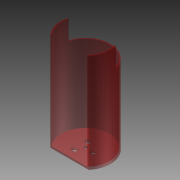
# Autodesk Inventor part: ss_inner_guide_top
Saved by Autodesk Inventor 2011 SP2 (Build 150309200, 309)
## iProperties
Created: 2012-05-22
Part Number: ss_inner_guide_top
Document SubType Name: Modeling
Designer: sungwook
Density: 1 g/cm^3
Author: sungwook
Autodesk Inventor part; units mm, degrees
ref_plane "YZ Plane" through (0, 0, 0) normal (1, 0, 0) x (0, 1, 0)
sketch "Sketch1" plane through (0, 0, 0) normal (0, 0, 1) x (1, 0, 0)
  circle A0 centre (0, 0) radius 12.75
  circle A1 centre (0, 0) radius 12.25
  dimension "d0" = 25.5
  dimension "d1" = 24.5
  constraints: 2 centre point, 2 coincident
  measures "d0" diameter of A0
  measures "d1" diameter of A1
extrude "Extrusion1" add sketch "Sketch1" along normal blind 49.5
sketch "Sketch2" plane through (0, 0, 49.5) normal (0, 0, 1) x (1, 0, 0)
  line L0 (-17.85, 0) -> (17.85, 0) projected
  line L1 (0, -17.85) -> (0, 17.85) projected
  line L2 (0, 0) -> (-12.3156, 3.2999)
  line L3 (0, 0) -> (-9.0156, -9.0156)
  line L4 (0, 0) -> (12.3156, 3.2999)
  line L5 (0, 0) -> (9.0156, -9.0156)
  arc A0 (11.8326, 3.1705) -> (-11.8326, 3.1705) centre (0, 0) ccw
  arc A1 (-8.6621, -8.6621) -> (8.6621, -8.6621) centre (0, 0) ccw
  circle A2 centre (0, 0) radius 12.75 projected
  dimension "d4" = 15
  dimension "d5" = 45
  constraints: 8 end point, 8 point on circle, 4 point on line, 2 centre point, 2 coincident, 2 symmetric about line
  measures "d4" angle of L0 L2
  measures "d5" angle of L3 L0
extrude "Extrusion2" cut sketch "Sketch2" against normal blind 10 contours L5 A1 L1 | L1 A1 L3 | A1 L5 A2 L1 | L1 A2 L3 A1 | A0 L2 A2 L1 | L1 A2 L4 A0
sketch "Sketch3" plane through (0, 0, 0) normal (0, 0, -1) x (-1, 0, 0)
  circle A0 centre (0, 0) radius 12.75 projected
extrude "Extrusion3" add sketch "Sketch3" along normal blind 1
ref_plane "Work Plane1" through (0, -12.75, 0) normal (0, 1, 0) x (-1, 0, 0)
ref_plane "Work Plane2" through (0, -12.75, 0) normal (0, 1, 0) x (-1, 0, 0)
sketch "Sketch7" plane through (0, 0, 49.5) normal (0, 0, 1) x (1, 0, 0)
  arc A0 (9.0156, -9.0156) -> (12.3156, 3.2999) centre (0, 0) ccw projected
  arc A1 (8.6621, -8.6621) -> (11.8326, 3.1705) centre (0, 0) ccw projected
  line L0 (8.6621, -8.6621) -> (9.0156, -9.0156) projected
  line L1 (-10.4211, -8.1317) -> (11.1081, -8.1317)
  line L2 (11.1081, -8.1317) -> (11.1081, -13.0652)
  line L3 (11.1081, -13.0652) -> (-10.4211, -13.0652)
  line L4 (-10.4211, -13.0652) -> (-10.4211, -8.1317)
  constraints: 8 end point, 2 parallel, 1 horizontal, 1 perpendicular
extrude "Extrusion6" cut sketch "Sketch7" against normal through all
sketch "Sketch9" plane through (0, 0, 0) normal (0, 0, 1) x (1, 0, 0)
  arc A0 (9.1617, -8.1317) -> (-9.1617, -8.1317) centre (0, 0) ccw projected
  line L0 (-17.85, 0) -> (17.85, 0) projected
  point P0 (4, 0)
  dimension "d29" = 4
  constraints: 1 point on line
  measures "d29" distance of point (4, 0) A0.centre
hole "Hole2" at (4, 0, 0) direction (0, 0, -1) diameter 1.778 depth 8 tip angle 118 countersink diameter 3.023 countersink angle 82 clearance for "Flat Head Machine Screw (82)" size "#0" standard "Ansi Unified Screw Threads"
pattern_circular "Circular Pattern1" count 3 over 360 about axis through (0, 0, -10) along (0, 0, 1) of "Hole2"
sketch "Sketch10" plane through (0, 0, 0) normal (0, 0, 1) x (1, 0, 0)
  arc A0 (9.1617, -8.1317) -> (-9.1617, -8.1317) centre (0, 0) ccw projected
hole "Hole3" at (0, 0, 0) direction (0, 0, -1) diameter 1.778 end through all
body "Solid1"
